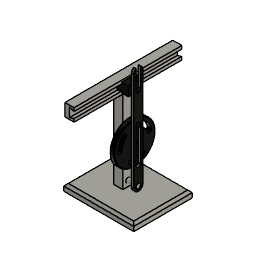
QuickReturnMechanism (Autodesk Fusion 360 design; units mm, degrees)
part number: 2026-03-23-03-57-25-303
part number: 2026-03-23-04-18-20-966
part number: 2026-03-23-04-23-05-528
part number: 2026-03-23-04-24-59-026
part number: 2026-03-23-04-43-20-055
Autodesk Fusion 360 part; units mm, degrees
note: some values were not read from the file. Chosen so that the rebuilt part matches the saved one: a direction.
sketch "Sketch1" plane through (0, 0, 0) normal (0, 1, 0) x (1, 0, 0)
  line L0 (61, -6) -> (-61, -6)
  line L1 (-61, -6) -> (-61, 6)
  line L2 (-61, 6) -> (61, 6)
  line L3 (61, 6) -> (61, -6)
  line L4 (61, -6) -> (-61, 6) construction
  line L5 (-61, -6) -> (61, 6) construction
  line L6 (0, -6) -> (-16, -6)
  line L7 (-16, -6) -> (-16, -172)
  line L8 (-16, -172) -> (0, -172)
  line L9 (0, -172) -> (0, -6)
  line L10 (0, -16) -> (18, -16)
  line L11 (18, -16) -> (18, -20)
  line L12 (18, -20) -> (0, -20)
  line L13 (0, -20) -> (0, -16)
  line L14 (0, -78) -> (12, -78)
  line L15 (12, -78) -> (12, -82)
  line L16 (12, -82) -> (0, -82)
  line L17 (0, -82) -> (0, -78)
  line L18 (0, -153) -> (12, -153)
  line L19 (12, -153) -> (12, -169)
  line L20 (12, -169) -> (0, -169)
  line L21 (0, -169) -> (0, -153)
  line L22 (-16, -150) -> (0, -150)
  line L23 (0, -161) -> (-8, -161) construction
  line L24 (-8, -161) -> (-8, -169)
  line L25 (-8, -169) -> (0, -166.4006)
  line L26 (-8, -153) -> (0, -155.5994)
  line L27 (-8, -161) -> (-8, -153)
  line L28 (12, -161) -> (18, -161)
  line L29 (18, -161) -> (18, -165)
  line L30 (18, -165) -> (12, -165)
  line L31 (12, -165) -> (12, -161)
  line L32 (12, -82) -> (4, -82)
  line L33 (4, -82) -> (4, -114)
  line L34 (4, -114) -> (12, -114)
  line L35 (12, -114) -> (12, -82)
  line L36 (12, -112) -> (18, -112)
  line L37 (18, -112) -> (18, -108)
  line L38 (18, -108) -> (12, -108)
  line L39 (12, -108) -> (12, -112)
  line L40 (18, -20) -> (18, -21.6178)
  dimension "d1" = 122
  dimension "d2" = 12
  dimension "d3" = 16
  dimension "d4" = 166
  dimension "d5" = 10
  dimension "d6" = 4
  dimension "d7" = 72
  dimension "d8" = 4
  dimension "d9" = 3
  dimension "d10" = 16
  dimension "d11" = 12
  dimension "d12" = -22
  dimension "d13" = 8
  dimension "d14" = 18
  dimension "d15" = 4
  dimension "d16" = 32
  dimension "d17" = 8
  dimension "d18" = 2
  dimension "d19" = 4
  dimension "d20" = 6
  constraint horizontal L0
  constraint perpendicular L0 L1
  constraint parallel L0 L2
  constraint parallel L1 L3
  constraint coincident L4 origin
  constraint coincident L5 origin
  constraint horizontal L6
  constraint vertical L7
  constraint horizontal L8
  constraint vertical L9
  constraint midpoint L0 L6.start
  constraint horizontal L10
  constraint vertical L11
  constraint horizontal L12
  constraint vertical L13
  constraint coincident L9 L10.start
  constraint horizontal L14
  constraint vertical L15
  constraint horizontal L16
  constraint vertical L17
  constraint coincident L9 L14.start
  constraint horizontal L18
  constraint vertical L19
  constraint horizontal L20
  constraint vertical L21
  constraint coincident L9 L18.start
  constraint midpoint L21 L23.start
  constraint perpendicular L21 L23
  constraint perpendicular L20 L24
  constraint coincident L9 L25.end
  constraint horizontal L20.end L24.end
  constraint symmetric L24.start L23 L27.start
  constraint symmetric L23 L24.end L26.start
  constraint symmetric L23 L25.end L26.end
  constraint horizontal L28
  constraint vertical L29
  constraint horizontal L30
  constraint vertical L31
  constraint midpoint L19 L28.start
  constraint horizontal L32
  constraint vertical L33
  constraint horizontal L34
  constraint vertical L35
  constraint horizontal L36
  constraint vertical L37
  constraint horizontal L38
  constraint vertical L39
  constraint coincident L35 L36.start
  constraint vertical L28.end L36.end
  constraint vertical L18.end L34.end
  constraint vertical L11.end L37.end
  constraint perpendicular L12 L40
  measures "d1" distance of L1.end L2.end
  measures "d2" distance of L0.end L1.end
  measures "d3" distance of L6.start L6.end
  measures "d4" distance of L6.start L8.end
  measures "d5" distance of L0 L10.end
  measures "d6" distance of L10.end L11.end
  measures "d7" distance of L0 L14.end
  measures "d8" distance of L14.end L15.end
  measures "d9" distance of L8.end L20
  measures "d10" distance of L18.end L19.end
  measures "d11" distance of L18.start L18.end
  measures "d13" distance of L23.start L23.end
  measures "d14" angle of L20 L25
  measures "d15" distance of L28.end L29.end
  measures "d16" distance of L32.end L33.end
  measures "d17" distance of L33.end L34.end
  measures "d18" distance of L34.end L36
  measures "d19" distance of L36.end L37.end
  measures "d20" distance of L28.start L28.end
extrude "Extrude1" add sketch "Sketch1" along normal mid plane 102 contours L0 L1 L2 L3 L6 makes body 1 in component "Base"
extrude "Extrude1'" add sketch "Sketch1" along normal mid plane 188 separate body contours L7 L8 L9 L21 L22 L24 L25 L26 L27 makes body 2
extrude "Extrude2" add sketch "Sketch1" along normal mid plane 18 contours L0 L6 L7 L9 L13 L17 L22 bodies 2
revolve "Revolve1" add sketch "Sketch1" angle 360 about axis through (0, 0, 16) along (1, 0, 0) contours L9 L10 L11 L12 L13 bodies 2
revolve "Revolve2" add sketch "Sketch1" angle 360 about axis through (0, 0, 78) along (1, 0, 0) contours L9 L14 L15 L16 L17 L32 bodies 2
extrude "Extrude1''" add sketch "Sketch1" along normal mid plane 22 separate body contours L9 L18 L19 L20 L21 L31 | L9 L21 L24 L25 L26 L27 makes body 3 in component "Slider"
revolve "Revolve1'" add sketch "Sketch1" angle 360 about axis through (12, 0, 161) along (1, 0, 0) contours L19 L28 L29 L30 L31 bodies 3 in component "Slider"
revolve "Revolve1''" add sketch "Sketch1" angle 360 about axis through (0, 0, 78) along (1, 0, 0) separate body contours L16 L32 L33 L34 L35 L39 makes body 4 in component "Disc"
revolve "Revolve2'" add sketch "Sketch1" angle 360 about axis through (18, 0, 108) along (-1, 0, 0) contours L35 L36 L37 L38 L39 bodies 4 in component "Disc"
sketch "Sketch2" plane through (12, 0, 0) normal (1, 0, 0) x (0, 1, 0)
  circle A0 centre (0, 108) radius 4
  circle A1 centre (0, 78) radius 4
  circle A2 centre (0, 78) radius 36
  arc A3 (-20.8398, 99.5802) -> (-30, 78) centre (0, 78) ccw
  arc A4 (-15.2825, 93.8255) -> (-20.8398, 99.5802) centre (-18.0611, 96.7028) ccw
  arc A5 (-15.2825, 93.8255) -> (-22, 78) centre (0, 78) ccw
  arc A6 (-30, 78) -> (-22, 78) centre (-26, 78) ccw
  arc A7 (-18.0611, 96.7028) -> (-26, 78) centre (0, 78) ccw construction
  line L0 (-18.0611, 96.7028) -> (0, 78) construction
  line L1 (0, 78) -> (-26, 78) construction
  dimension "d34" = 46
  dimension "d35" = 4
  dimension "d36" = 26
  constraint tangent A3 A4
  constraint tangent A4 A5
  constraint tangent A5 A6
  constraint tangent A3 A6
  constraint coincident A1.centre A2.centre
  constraint coincident A4.centre A7.start
  constraint coincident A6.centre A7.end
  constraint horizontal L1
  measures "d34" angle of L0 L1
  measures "d35" radius of A4
  measures "d36" radius of A7
extrude "Extrude1'''" cut sketch "Sketch2" against normal through all contours A3 A4 A5 A6 bodies 4 in component "Disc"
pattern_circular "C-Pattern1" count 3 over 360 about axis through (12, 0, 78) along (-1, 0, 0) of "Extrude1'''" in component "Disc"
chamfer "Chamfer1" distance 1 angle 45 1 faces at (6.6667, 1.7945, 113.9552) on bodies 4 in component "Disc"
chamfer "Chamfer1'" distance 4 angle 45 1 faces at (20.3333, 17, 6) on bodies 1 in component "Base"
sketch "Sketch3" plane through (18, 0, 0) normal (1, 0, 0) x (0, 1, 0)
  circle A0 centre (0, 16) radius 4
  line L0 (8, 16) -> (8, 188)
  arc A1 (8, 188) -> (-8, 188) centre (0, 188) ccw
  line L1 (-8, 188) -> (-8, 16)
  arc A2 (-8, 16) -> (8, 16) centre (0, 16) ccw
  line L2 (0, 16) -> (0, 188) construction
  circle A3 centre (0, 16) radius 4
  circle A4 centre (0, 78) radius 4
  circle A5 centre (0, 108) radius 4
  circle A6 centre (0, 161) radius 4
  line L3 (-4, 108) -> (-4, 48)
  arc A7 (-4, 48) -> (4, 48) centre (0, 48) ccw
  line L4 (4, 48) -> (4, 108)
  arc A8 (4, 108) -> (-4, 108) centre (0, 108) ccw
  line L5 (0, 108) -> (0, 48) construction
  line L6 (4, 161) -> (4, 196)
  arc A9 (4, 196) -> (-4, 196) centre (0, 196) ccw
  line L7 (-4, 196) -> (-4, 161)
  arc A10 (-4, 161) -> (4, 161) centre (0, 161) ccw
  line L8 (0, 161) -> (0, 196) construction
  dimension "d42" = 172
  dimension "d43" = 8
  dimension "d44" = 60
  constraint tangent L0 A1
  constraint tangent A1 L1
  constraint parallel L0 L1
  constraint tangent L1 A2
  constraint tangent L0 A2
  constraint vertical L2
  constraint coincident A0.centre A2.centre
  constraint tangent L3 A7
  constraint tangent A7 L4
  constraint parallel L3 L4
  constraint tangent L4 A8
  constraint tangent L3 A8
  constraint parallel L2 L5
  constraint coincident A5.centre A8.centre
  constraint equal A5 A8
  constraint tangent L6 A9
  constraint tangent A9 L7
  constraint parallel L6 L7
  constraint tangent L7 A10
  constraint tangent L6 A10
  constraint parallel L2 L8
  constraint coincident A6.centre A10.centre
  constraint equal A6 A10
  constraint coincident A1 A9.centre
  measures "d42" distance of A0.centre A1.centre
  measures "d43" radius of A1
  measures "d44" distance of A5.centre A7.centre
extrude "Extrude1''''" add sketch "Sketch3" against normal blind 4 separate body contours L0 A1 L1 A2 A6 L6 L7 A10 makes body 5 in component "Crank"
other "GeometricRelationship1"
other "GeometricRelationship2"
component "Base" placed x (1, 0, 0) y (0, 1, 0) z (0, 0, 1) at (0, 0, 0)
component "Slider" placed x (1, 0, 0) y (0, 1, 0) z (0, 0, 1) at (0, 0, 0)
component "Disc" placed x (1, 0, 0) y (0, 1, 0) z (0, 0, 1) at (0, 0, 0)
component "Crank" placed x (1, 0, 0) y (0, 1, 0) z (0, 0, 1) at (0, 0, 0)
